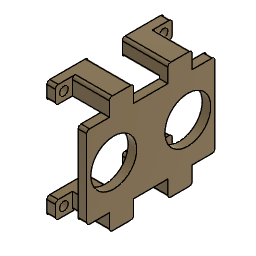
Base Sensor Hueco 2.0 v6 v7 v2 (Autodesk Fusion 360 design; units mm, degrees)
Autodesk Fusion 360 part; units mm, degrees
note: some values were not read from the file. Chosen so that the rebuilt part matches the saved one: which bodies a step acts on. Set by a fixed rule: which sketch regions a step uses.
sketch "Boceto1" plane through (0, 0, 0) normal (0, 0, 1) x (1, 0, 0)
  line L0 (-22.5, -25.5) -> (22.5, -25.5)
  line L1 (22.5, -25.5) -> (22.5, 25.5)
  line L2 (22.5, 25.5) -> (-22.5, 25.5)
  line L3 (-22.5, 25.5) -> (-22.5, -25.5)
  line L4 (-22.5, -25.5) -> (22.5, 25.5) construction
  line L5 (22.5, -25.5) -> (-22.5, 25.5) construction
  dimension "d15" = 45
  dimension "d16" = 51
  constraint horizontal L0
  constraint perpendicular L0 L1
  constraint parallel L0 L2
  constraint parallel L1 L3
  constraint coincident L4 origin
  constraint coincident L5 origin
  measures "d15" distance of L1.end L2.end
  measures "d16" distance of L0.end L1.end
extrude "Extruir4" add sketch "Boceto1" along normal mid plane 3 makes body 1
sketch "Boceto4" plane through (0, 0, 0) normal (0, 1, 0) x (1, 0, 0)
  line L0 (0, 22.5) -> (3, 22.5)
  line L1 (3, 22.5) -> (3, -22.5)
  line L2 (3, -22.5) -> (0, -22.5)
  line L3 (0, -22.5) -> (0, 22.5)
  line L4 (3, -14.5) -> (13, -14.5)
  line L5 (13, -14.5) -> (13, -11.5)
  line L6 (13, -11.5) -> (3, -11.5)
  line L7 (3, -11.5) -> (3, -14.5)
  line L8 (13, -14.5) -> (16, -14.5)
  line L9 (16, -14.5) -> (16, -8.5)
  line L10 (16, -8.5) -> (13, -8.5)
  line L11 (13, -8.5) -> (13, -14.5)
  line L12 (1.75, 0) -> (22.5, 0)
  line L13 (13, 11.5) -> (3, 11.5)
  line L14 (3, 14.5) -> (13, 14.5)
  line L15 (13, 14.5) -> (13, 11.5)
  line L16 (13, 14.5) -> (16, 14.5)
  line L17 (16, 14.5) -> (16, 8.5)
  line L18 (16, 8.5) -> (13, 8.5)
  line L19 (13, 8.5) -> (13, 14.5)
  line L20 (3, 11.5) -> (3, 14.5)
  dimension "d21" = 3
  dimension "d22" = 45
  dimension "d23" = 22.5
  dimension "d24" = 10
  dimension "d25" = 3
  dimension "d26" = 11.5
  dimension "d27" = 3
  dimension "d28" = 6
  constraint horizontal L0
  constraint vertical L1
  constraint horizontal L2
  constraint vertical L3
  constraint coincident origin L3
  constraint horizontal L4
  constraint vertical L5
  constraint horizontal L6
  constraint vertical L7
  constraint coincident L1 L4.start
  constraint horizontal L8
  constraint vertical L9
  constraint horizontal L10
  constraint vertical L11
  constraint symmetric L4.start L12 L14.start
  constraint symmetric L4.end L12 L14.end
  constraint symmetric L5.end L12 L13.start
  constraint symmetric L6.end L12 L13.end
  constraint symmetric L8.end L12 L16.end
  constraint symmetric L9.end L12 L17.end
  constraint symmetric L10.end L12 L18.end
  measures "d21" distance of L0.start L0.end
  measures "d22" distance of L0.start L2.end
  measures "d23" distance of origin L0
  measures "d24" distance of L4.start L4.end
  measures "d25" distance of L4.start L6.end
  measures "d26" distance of origin L6
  measures "d27" distance of L4.end L8.end
  measures "d28" distance of L4.end L10.end
extrude "Extruir5" add sketch "Boceto4" along normal mid plane 45 separate body makes body 2
sketch "Boceto5" plane through (3, 0, 0) normal (1, 0, 0) x (0, 1, 0)
  line L0 (-22.5, 14.5) -> (22.5, 14.5)
  line L1 (22.5, 14.5) -> (22.5, 22.5)
  line L2 (22.5, 22.5) -> (-22.5, 22.5)
  line L3 (-22.5, 22.5) -> (-22.5, 14.5)
  circle A0 centre (-17.5, 17.5) radius 1.5
  circle A1 centre (17.5, 17.5) radius 1.5
  circle A2 centre (-17.5, -17.5) radius 1.5
  circle A3 centre (17.5, -17.5) radius 1.5
  dimension "d31" = 3
  dimension "d32" = 3
  dimension "d33" = 3
  dimension "d34" = 3
  dimension "d35" = 17.5
  dimension "d36" = 35
  dimension "d37" = 35
  dimension "d38" = 17.5
  constraint horizontal A0.centre A1.centre
  constraint horizontal A2.centre A3.centre
  constraint vertical A0.centre A2.centre
  constraint vertical A1.centre A3.centre
  measures "d31" diameter of A0
  measures "d32" diameter of A1
  measures "d33" diameter of A2
  measures "d34" diameter of A3
  measures "d35" vertical distance of origin A0.centre
  measures "d36" distance of A0.centre A2.centre
  measures "d37" distance of A0.centre A1.centre
  measures "d38" horizontal distance of origin A0.centre
extrude "Extruir6" cut sketch "Boceto5" against normal blind 3 contours A0 | A1 | A2 | A3 bodies 2
sketch "Boceto6" plane through (0, 0, -14.5) normal (0, 0, -1) x (1, 0, 0)
  line L0 (3, 22.5) -> (3, -22.5)
  line L1 (3, -22.5) -> (16, -22.5)
  line L2 (16, -22.5) -> (16, 22.5)
  line L3 (16, 22.5) -> (3, 22.5)
  line L4 (3, 6) -> (16, 6)
  line L5 (16, 6) -> (16, -6)
  line L6 (16, -6) -> (3, -6)
  line L7 (3, -6) -> (3, 6)
  dimension "d41" = 12
  dimension "d42" = 6
  constraint horizontal L4
  constraint vertical L5
  constraint horizontal L6
  constraint vertical L7
  constraint coincident L2 L5.end
  constraint coincident L0 L4.start
  measures "d41" distance of L4.start L6.end
  measures "d42" distance of origin L6
extrude "Extruir7" cut sketch "Boceto6" against normal blind 29 contours L0 L2 L4 L5 L6 L7 bodies 2
sketch "Sketch7" plane through (3, 0, 0) normal (1, 0, 0) x (0, 1, 0)
  circle A0 centre (17.5, 17.5) radius 1.5
  circle A1 centre (-17.5, 17.5) radius 1.5
  circle A2 centre (17.5, -17.5) radius 1.5
  circle A3 centre (-17.5, -17.5) radius 1.5
  line L0 (-22.5, -22.5) -> (22.5, -22.5)
  line L1 (22.5, -22.5) -> (22.5, -14.5)
  line L2 (22.5, -14.5) -> (6, -14.5)
  line L3 (6, -14.5) -> (6, -11.5)
  line L4 (6, -11.5) -> (22.5, -11.5)
  line L5 (22.5, -11.5) -> (22.5, 11.5)
  line L6 (22.5, 11.5) -> (6, 11.5)
  line L7 (6, 11.5) -> (6, 14.5)
  line L8 (6, 14.5) -> (22.5, 14.5)
  line L9 (22.5, 14.5) -> (22.5, 22.5)
  line L10 (22.5, 22.5) -> (-22.5, 22.5)
  line L11 (-22.5, 22.5) -> (-22.5, 14.5)
  line L12 (-22.5, 14.5) -> (-6, 14.5)
  line L13 (-6, 14.5) -> (-6, 11.5)
  line L14 (-6, 11.5) -> (-22.5, 11.5)
  line L15 (-22.5, 11.5) -> (-22.5, -11.5)
  line L16 (-22.5, -11.5) -> (-6, -11.5)
  line L17 (-6, -11.5) -> (-6, -14.5)
  line L18 (-6, -14.5) -> (-22.5, -14.5)
  line L19 (-22.5, -14.5) -> (-22.5, -22.5)
  line L20 (-14.5, 20.5) -> (-20.5, 20.5)
  line L21 (-20.5, 20.5) -> (-20.5, 14.5)
  line L22 (-20.5, 14.5) -> (-14.5, 14.5)
  line L23 (-14.5, 14.5) -> (-14.5, 20.5)
  line L24 (-14.5, 20.5) -> (-20.5, 14.5) construction
  line L25 (-20.5, 20.5) -> (-14.5, 14.5) construction
  line L26 (20.5, 14.5) -> (14.5, 14.5)
  line L27 (14.5, 14.5) -> (14.5, 20.5)
  line L28 (14.5, 20.5) -> (20.5, 20.5)
  line L29 (20.5, 20.5) -> (20.5, 14.5)
  line L30 (20.5, 14.5) -> (14.5, 20.5) construction
  line L31 (14.5, 14.5) -> (20.5, 20.5) construction
  line L32 (-20.5, -20.5) -> (-14.5, -20.5)
  line L33 (-14.5, -20.5) -> (-14.5, -14.5)
  line L34 (-14.5, -14.5) -> (-20.5, -14.5)
  line L35 (-20.5, -14.5) -> (-20.5, -20.5)
  line L36 (-20.5, -20.5) -> (-14.5, -14.5) construction
  line L37 (-14.5, -20.5) -> (-20.5, -14.5) construction
  line L38 (20.5, -20.5) -> (14.5, -20.5)
  line L39 (14.5, -20.5) -> (14.5, -14.5)
  line L40 (14.5, -14.5) -> (20.5, -14.5)
  line L41 (20.5, -14.5) -> (20.5, -20.5)
  line L42 (20.5, -20.5) -> (14.5, -14.5) construction
  line L43 (14.5, -20.5) -> (20.5, -14.5) construction
  line L44 (-20.5, 20.5) -> (-26, 20.5)
  line L45 (-20.5, 14.5) -> (-26, 14.5)
  line L46 (-26, 14.5) -> (-26, 20.5)
  line L47 (-20.5, -14.5) -> (-26.5, -14.5)
  line L48 (-26.5, -14.5) -> (-26.5, -20.5)
  line L49 (-26.5, -20.5) -> (-20.5, -20.5)
  line L50 (-20.5, -20.5) -> (-20.5, -14.5)
  line L51 (20.5, 20.5) -> (26.5, 20.5)
  line L52 (26.5, 20.5) -> (26.5, 14.5)
  line L53 (26.5, 14.5) -> (20.5, 14.5)
  line L54 (20.5, 14.5) -> (20.5, 20.5)
  line L55 (20.5, -14.5) -> (26.5, -14.5)
  line L56 (26.5, -14.5) -> (26.5, -20.5)
  line L57 (26.5, -20.5) -> (20.5, -20.5)
  line L58 (20.5, -20.5) -> (20.5, -14.5)
  point P0 (-17.5, 17.5)
  point P1 (17.5, 17.5)
  point P2 (-17.5, -17.5)
  point P3 (17.5, -17.5)
  dimension "d45" = 6
  dimension "d46" = 6
  dimension "d47" = 6
  dimension "d48" = 6
  dimension "d49" = 6
  dimension "d50" = 6
  dimension "d51" = 6
  dimension "d52" = 6
  dimension "d53" = 6
  dimension "d54" = 6
  dimension "d55" = 6
  dimension "d56" = 6
  dimension "d57" = 6
  dimension "d58" = 6
  constraint horizontal L20
  constraint perpendicular L20 L21
  constraint parallel L20 L22
  constraint parallel L21 L23
  constraint coincident L24 P0
  constraint coincident L25 P0
  constraint coincident P0 A1.centre
  constraint horizontal L26
  constraint perpendicular L26 L27
  constraint parallel L26 L28
  constraint parallel L27 L29
  constraint coincident L30 P1
  constraint coincident L31 P1
  constraint coincident A0.centre P1
  constraint horizontal L32
  constraint perpendicular L32 L33
  constraint parallel L32 L34
  constraint parallel L33 L35
  constraint coincident L36 P2
  constraint coincident L37 P2
  constraint coincident P2 A3.centre
  constraint horizontal L38
  constraint perpendicular L38 L39
  constraint parallel L38 L40
  constraint parallel L39 L41
  constraint coincident L42 P3
  constraint coincident L43 P3
  constraint coincident A2.centre P3
  constraint perpendicular L21 L44
  constraint perpendicular L21 L45
  constraint perpendicular L44 L46
  constraint horizontal L47
  constraint vertical L48
  constraint horizontal L49
  constraint vertical L50
  constraint horizontal L51
  constraint vertical L52
  constraint horizontal L53
  constraint vertical L54
  constraint horizontal L55
  constraint vertical L56
  constraint horizontal L57
  constraint vertical L58
  measures "d45" distance of L21.end L22.end
  measures "d46" distance of L20.end L21.end
  measures "d47" distance of L27.end L28.end
  measures "d48" distance of L26.end L27.end
  measures "d49" distance of L33.end L34.end
  measures "d50" distance of L32.end L33.end
  measures "d51" distance of L39.end L40.end
  measures "d52" distance of L38.end L39.end
  measures "d53" distance of L34.end L47.end
  measures "d54" distance of L34.end L32.start
  measures "d55" distance of L28.end L51.end
  measures "d56" distance of L28.end L26.start
  measures "d57" distance of L40.end L55.end
  measures "d58" distance of L40.end L38.start
extrude "Extrude8" add sketch "Sketch7" along normal blind 3 separate body contours L8 L26 L27 L28 L29 L54 makes body 3
extrude "Extrude9" add sketch "Sketch7" along normal blind 3 separate body contours L12 L20 L21 L22 L23 makes body 4
extrude "Extrude10" add sketch "Sketch7" along normal blind 3 separate body contours L18 L32 L33 L34 L35 L50 makes body 5
extrude "Extrude11" add sketch "Sketch7" along normal blind 3 separate body contours L2 L38 L39 L40 L41 L58 makes body 6
sketch "Sketch8" plane through (3, 0, 0) normal (1, 0, 0) x (0, 1, 0)
sketch "Sketch9" plane through (0, 0, 0) normal (1, 0, 0) x (0, 1, 0)
sketch "Sketch10" plane through (0, 0, 0) normal (1, 0, 0) x (0, 1, 0)
sketch "Sketch11" plane through (6, 0, 0) normal (1, 0, 0) x (0, 1, 0)
  circle A0 centre (-17.5, 17.5) radius 1.5
  line L0 (-14.5, 14.5) -> (-14.5, 20.5)
  line L1 (-14.5, 20.5) -> (-20.5, 20.5)
  line L2 (-20.5, 20.5) -> (-20.5, 14.5)
  line L3 (-20.5, 14.5) -> (-14.5, 14.5)
  line L4 (-14.5, 20.5) -> (-6, 20.5)
  line L5 (-6, 20.5) -> (-6, 14.5)
  line L6 (-6, 14.5) -> (-14.5, 14.5)
  line L7 (-14.5, 14.5) -> (-14.5, 20.5)
  dimension "d67" = 8.5
  dimension "d68" = 6
  constraint horizontal L4
  constraint vertical L5
  constraint horizontal L6
  constraint vertical L7
  constraint coincident L0.end L1.start
  measures "d67" distance of L0.end L4.end
  measures "d68" distance of L0.end L0.start
sketch "Sketch12" plane through (6, 0, 0) normal (1, 0, 0) x (0, 1, 0)
  circle A0 centre (-17.5, -17.5) radius 1.5
  line L0 (-14.5, -20.5) -> (-14.5, -14.5)
  line L1 (-14.5, -14.5) -> (-20.5, -14.5)
  line L2 (-20.5, -14.5) -> (-20.5, -20.5)
  line L3 (-20.5, -20.5) -> (-14.5, -20.5)
  line L4 (-14.5, -14.5) -> (-6, -14.5)
  line L5 (-6, -14.5) -> (-6, -20.5)
  line L6 (-6, -20.5) -> (-14.5, -20.5)
  line L7 (-14.5, -20.5) -> (-14.5, -14.5)
  dimension "d69" = 8.5
  dimension "d70" = 6
  constraint horizontal L4
  constraint vertical L5
  constraint horizontal L6
  constraint vertical L7
  constraint coincident L0.end L1.start
  measures "d69" distance of L0.end L4.end
  measures "d70" distance of L0.end L0.start
sketch "Sketch13" plane through (6, 0, 0) normal (1, 0, 0) x (0, 1, 0)
  circle A0 centre (17.5, -17.5) radius 1.5
  line L0 (14.5, -20.5) -> (20.5, -20.5)
  line L1 (20.5, -20.5) -> (20.5, -14.5)
  line L2 (20.5, -14.5) -> (14.5, -14.5)
  line L3 (14.5, -14.5) -> (14.5, -20.5)
  line L4 (14.5, -14.5) -> (6, -14.5)
  line L5 (6, -14.5) -> (6, -20.5)
  line L6 (6, -20.5) -> (14.5, -20.5)
  line L7 (14.5, -20.5) -> (14.5, -14.5)
  dimension "d71" = 8.5
  dimension "d72" = 6
  constraint horizontal L4
  constraint vertical L5
  constraint horizontal L6
  constraint vertical L7
  constraint coincident L2.end L3.start
  measures "d71" distance of L2.end L4.end
  measures "d72" distance of L2.end L0.start
sketch "Sketch14" plane through (6, 0, 0) normal (1, 0, 0) x (0, 1, 0)
  circle A0 centre (17.5, 17.5) radius 1.5
  line L0 (14.5, 14.5) -> (20.5, 14.5)
  line L1 (20.5, 14.5) -> (20.5, 20.5)
  line L2 (20.5, 20.5) -> (14.5, 20.5)
  line L3 (14.5, 20.5) -> (14.5, 14.5)
  line L4 (14.5, 20.5) -> (6, 20.5)
  line L5 (6, 20.5) -> (6, 14.5)
  line L6 (6, 14.5) -> (14.5, 14.5)
  line L7 (14.5, 14.5) -> (14.5, 20.5)
  dimension "d73" = 8.5
  dimension "d74" = 6
  constraint horizontal L4
  constraint vertical L5
  constraint horizontal L6
  constraint vertical L7
  constraint coincident L2.end L3.start
  measures "d73" distance of L2.end L4.end
  measures "d74" distance of L2.end L0.start
extrude "Extrude12" add sketch "Sketch12" sketch "Sketch11" sketch "Sketch13" sketch "Sketch14" along normal blind 10 and the other way blind 3 separate body contours L0 L4 L5 L6 L7 of sketch 2 contours L0 L4 L5 L6 L7 of sketch 3 contours L3 L4 L5 L6 L7 of sketch 4 contours L3 L4 L5 L6 L7 makes body 7 at (11.6667, 8.8333, -14.5) makes body 8 at (11.6667, -11.6667, -20.5) makes body 9 at (11.6667, -11.6667, 14.5) makes body 10 at (11.6667, 8.8333, 20.5)
extrude "Extrude13" add 4 faces at (16, -8.8333, 16.5) (16, 11.6667, 18.5) (16, 11.6667, -18.5) (16, -11.6667, -18.5) along direction (1, 0, 0) blind 3 separate body on bodies 7 8 9 10 makes body 11 at (16, 11.6667, -18.5) makes body 12 at (16, -8.8333, 16.5) makes body 13 at (16, 11.6667, 18.5) makes body 14 at (16, -11.6667, -18.5)
combine "Combine1" operation add target body 10 tool bodies 13
combine "Combine2" operation add target body 7 tool bodies 11 8 14 9 12 10 makes body 15 at (13.6667, -11.6667, -14.5) makes body 16 at (13.6667, -11.6667, 20.5) makes body 17 at (13.6667, 11.6667, 20.5)
sketch "Sketch15" plane through (16, 0, 0) normal (1, 0, 0) x (0, 1, 0)
  line L0 (-6, 14.5) -> (-22.5, 14.5)
  line L1 (-22.5, 14.5) -> (-22.5, 8.5)
  line L2 (-22.5, 14.5) -> (22.5, 14.5)
  line L3 (22.5, 14.5) -> (22.5, -15.5)
  line L4 (22.5, -15.5) -> (-22.5, -15.5)
  line L5 (-22.5, -15.5) -> (-22.5, 14.5)
  dimension "d81" = 45
  dimension "d82" = 30
  constraint horizontal L2
  constraint vertical L3
  constraint horizontal L4
  constraint vertical L5
  constraint coincident L0.end L1.start
  measures "d81" distance of L0.end L2.end
  measures "d82" distance of L0.end L4.end
extrude "Extrude14" add sketch "Sketch15" along normal blind 3 separate body makes body 18
extrude "Extrude15" cut 1 faces at (18, 7.5, -15.5) along direction (0, 0, 1) blind 1 on bodies 18 bodies 7 15 18
extrude "Extrude16" add 1 faces at (16, -8.8333, -15.1667) along direction (1, 0, 0) blind 3 separate body on bodies 15 makes body 19
extrude "Extrude17" add 1 faces at (16, 11.6667, -15.1667) along direction (1, 0, 0) blind 3 separate body on bodies 7 makes body 20
combine "Combine3" operation add target body 15 tool bodies 19
combine "Combine4" operation add target body 7 tool bodies 20
combine "Combine5" operation add target body 4 tool bodies 16 18 15 7 6 5 17 3
fillet "Fillet1" radius 1 1 edges at (4.5, -20.5, -20.5) on bodies 4
fillet "Fillet2" radius 1 3 edges at (4.5, -20.5, 14.5) (17.5, -22.5, 14.5) (17.5, -22.5, -14.5) on bodies 4
fillet "Fillet3" radius 1 2 edges at (4.5, -20.5, -14.5) (4.5, -20.5, 20.5) on bodies 4
fillet "Fillet4" radius 1 6 edges at (4.5, 20.5, -20.5) (4.5, 20.5, -14.5) (17.5, 22.5, -14.5) (17.5, 22.5, 14.5) (4.5, 20.5, 14.5) (4.5, 20.5, 20.5) on bodies 4
fillet "Fillet5" radius 1 2 edges at (12.5, 14.5, 20.5) (11, 6, 20.5) on bodies 4
fillet "Fillet6" radius 1 2 edges at (11, -6, 20.5) (12.5, -14.5, 20.5) on bodies 4
fillet "Fillet7" radius 1 4 edges at (12.5, 14.5, -20.5) (11, 6, -20.5) (11, -6, -20.5) (12.5, -14.5, -20.5) on bodies 4
fillet "Fillet8" radius 1 4 edges at (9.5, 6, 14.5) (9.5, -6, 14.5) (9.5, -6, -14.5) (9.5, 6, -14.5) on bodies 4
sketch "Sketch16" plane through (19, 0, 0) normal (1, 0, 0) x (0, 1, 0)
  arc A0 (-14.5, -19.5) -> (-13.5, -20.5) centre (-13.5, -19.5) ccw
  line L0 (-13.5, -20.5) -> (-7, -20.5)
  arc A1 (-7, -20.5) -> (-6, -19.5) centre (-7, -19.5) ccw
  line L1 (-6, -19.5) -> (-6, -14.5)
  line L2 (-6, -14.5) -> (6, -14.5)
  line L3 (6, -14.5) -> (6, -19.5)
  arc A2 (6, -19.5) -> (7, -20.5) centre (7, -19.5) ccw
  line L4 (7, -20.5) -> (13.5, -20.5)
  arc A3 (13.5, -20.5) -> (14.5, -19.5) centre (13.5, -19.5) ccw
  line L5 (14.5, -19.5) -> (14.5, -14.5)
  line L6 (14.5, -14.5) -> (21.5, -14.5)
  arc A4 (21.5, -14.5) -> (22.5, -13.5) centre (21.5, -13.5) ccw
  line L7 (22.5, -13.5) -> (22.5, 13.5)
  arc A5 (22.5, 13.5) -> (21.5, 14.5) centre (21.5, 13.5) ccw
  line L8 (21.5, 14.5) -> (14.5, 14.5)
  line L9 (14.5, 14.5) -> (14.5, 19.5)
  arc A6 (14.5, 19.5) -> (13.5, 20.5) centre (13.5, 19.5) ccw
  line L10 (13.5, 20.5) -> (7, 20.5)
  arc A7 (7, 20.5) -> (6, 19.5) centre (7, 19.5) ccw
  line L11 (6, 19.5) -> (6, 14.5)
  line L12 (6, 14.5) -> (-6, 14.5)
  line L13 (-6, 14.5) -> (-6, 19.5)
  arc A8 (-6, 19.5) -> (-7, 20.5) centre (-7, 19.5) ccw
  line L14 (-7, 20.5) -> (-13.5, 20.5)
  arc A9 (-13.5, 20.5) -> (-14.5, 19.5) centre (-13.5, 19.5) ccw
  line L15 (-14.5, 19.5) -> (-14.5, 14.5)
  line L16 (-14.5, 14.5) -> (-21.5, 14.5)
  arc A10 (-21.5, 14.5) -> (-22.5, 13.5) centre (-21.5, 13.5) ccw
  line L17 (-22.5, 13.5) -> (-22.5, -13.5)
  arc A11 (-22.5, -13.5) -> (-21.5, -14.5) centre (-21.5, -13.5) ccw
  line L18 (-21.5, -14.5) -> (-14.5, -14.5)
  line L19 (-14.5, -14.5) -> (-14.5, -19.5)
  circle A12 centre (-10, 0) radius 5
  circle A13 centre (10, 0) radius 5
  dimension "d107" = 10
  measures "d107" diameter of A13
extrude "Extrude18" cut sketch "Sketch16" against normal blind 10 contours A12 | A13 bodies 4
extrude "Extrude19" add sketch "Sketch16" against normal blind 3 contours A12 | A13 bodies 4
sketch "Sketch17" plane through (19, 0, 0) normal (1, 0, 0) x (0, 1, 0)
  arc A0 (-14.5, -19.5) -> (-13.5, -20.5) centre (-13.5, -19.5) ccw
  line L0 (-13.5, -20.5) -> (-7, -20.5)
  arc A1 (-7, -20.5) -> (-6, -19.5) centre (-7, -19.5) ccw
  line L1 (-6, -19.5) -> (-6, -14.5)
  line L2 (-6, -14.5) -> (6, -14.5)
  line L3 (6, -14.5) -> (6, -19.5)
  arc A2 (6, -19.5) -> (7, -20.5) centre (7, -19.5) ccw
  line L4 (7, -20.5) -> (13.5, -20.5)
  arc A3 (13.5, -20.5) -> (14.5, -19.5) centre (13.5, -19.5) ccw
  line L5 (14.5, -19.5) -> (14.5, -14.5)
  line L6 (14.5, -14.5) -> (21.5, -14.5)
  arc A4 (21.5, -14.5) -> (22.5, -13.5) centre (21.5, -13.5) ccw
  line L7 (22.5, -13.5) -> (22.5, 13.5)
  arc A5 (22.5, 13.5) -> (21.5, 14.5) centre (21.5, 13.5) ccw
  line L8 (21.5, 14.5) -> (14.5, 14.5)
  line L9 (14.5, 14.5) -> (14.5, 19.5)
  arc A6 (14.5, 19.5) -> (13.5, 20.5) centre (13.5, 19.5) ccw
  line L10 (13.5, 20.5) -> (7, 20.5)
  arc A7 (7, 20.5) -> (6, 19.5) centre (7, 19.5) ccw
  line L11 (6, 19.5) -> (6, 14.5)
  line L12 (6, 14.5) -> (-6, 14.5)
  line L13 (-6, 14.5) -> (-6, 19.5)
  arc A8 (-6, 19.5) -> (-7, 20.5) centre (-7, 19.5) ccw
  line L14 (-7, 20.5) -> (-13.5, 20.5)
  arc A9 (-13.5, 20.5) -> (-14.5, 19.5) centre (-13.5, 19.5) ccw
  line L15 (-14.5, 19.5) -> (-14.5, 14.5)
  line L16 (-14.5, 14.5) -> (-21.5, 14.5)
  arc A10 (-21.5, 14.5) -> (-22.5, 13.5) centre (-21.5, 13.5) ccw
  line L17 (-22.5, 13.5) -> (-22.5, -13.5)
  arc A11 (-22.5, -13.5) -> (-21.5, -14.5) centre (-21.5, -13.5) ccw
  line L18 (-21.5, -14.5) -> (-14.5, -14.5)
  line L19 (-14.5, -14.5) -> (-14.5, -19.5)
  line L20 (5, -3) -> (-5, -3)
  line L21 (-5, -3) -> (-5, 3)
  line L22 (-5, 3) -> (5, 3)
  line L23 (5, 3) -> (5, -3)
  line L24 (5, -3) -> (-5, 3) construction
  line L25 (-5, -3) -> (5, 3) construction
  line L26 (5, 0) -> (13, 0)
  line L27 (-5, 0) -> (-13, 0)
  circle A12 centre (-13, 0) radius 8
  dimension "d112" = 10
  dimension "d113" = 8
  dimension "d115" = 16
  constraint horizontal L20
  constraint perpendicular L20 L21
  constraint parallel L20 L22
  constraint parallel L21 L23
  constraint coincident L24 origin
  constraint coincident L25 origin
  constraint midpoint L23 L26.start
  constraint perpendicular L23 L26
  constraint midpoint L21 L27.start
  constraint perpendicular L21 L27
  constraint coincident L27.end A12.centre
  measures "d112" distance of L21.end L22.end
  measures "d113" distance of L27.start L27.end
  measures "d115" diameter of A12
extrude "Extrude20" cut sketch "Sketch17" against normal blind 44 contours A12 bodies 4
extrude "Extrude21" add sketch "Sketch17" against normal blind 3 contours A12 bodies 4
sketch "Sketch18" plane through (19, 0, 0) normal (1, 0, 0) x (0, 1, 0)
  circle A0 centre (-13, 0) radius 8.05
  circle A1 centre (13, 0) radius 8.05
  dimension "d120" = 16.1
  dimension "d121" = 16.1
  measures "d120" diameter of A0
  measures "d121" diameter of A1
extrude "Extrude22" cut sketch "Sketch18" against normal blind 10 bodies 4
hidden bodies 1 2
equation "d23 = ( 45 / 2 ) * 1 mm"
equation "d26 = ( 23 / 2 ) * 1 mm"
equation "d35 = ( 35 / 2 ) * 1 mm"
equation "d38 = ( 35 / 2 ) * 1 mm"
